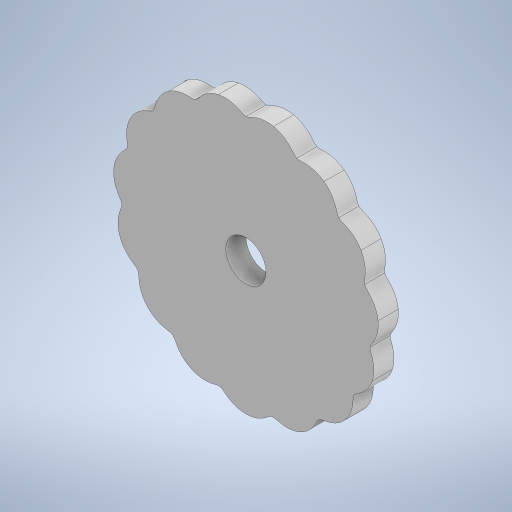
# Autodesk Inventor part: 사이클로이드 기어 001
Saved by Autodesk Inventor 2023 (Build 270158000, 158)
## iProperties
Created: 2022-06-19
Part Number: 사이클로이드 기어 001
Material: 일반
Document SubType Name: Modeling
Designer: fly01
Density: 1 g/cm^3
Appearance: 기본값
Author: fly01
Autodesk Inventor part; units mm, degrees
ref_plane "YZ Plane" through (0, 0, 0) normal (1, 0, 0) x (0, 1, 0)
ref_plane "XZ Plane" through (0, 0, 0) normal (0, 1, 0) x (-1, 0, 0)
ref_plane "XY Plane" through (0, 0, 0) normal (0, 0, 1) x (1, 0, 0)
sketch "스케치3" plane through (0, 0, 0) normal (0, 0, 1) x (1, 0, 0)
  circle A0 centre (0, 0) radius 30 construction
  circle A1 centre (-6.6532, 31.3007) radius 2 construction
  line L0 (-6.6532, 31.3007) -> (0, 0)
  line L1 (-6.6532, 31.3007) -> (-6.8611, 32.2789)
  line L2 (0, 30) -> (0, 0) construction
  spline S0 degree 4 poles (-6.8611, 32.2789) (-6.5216, 32.351) (-6.042, 32.4243) (-5.4252, 32.4676) (-4.6868, 32.4443) (-4.17, 32.3935) (-3.6752, 32.3125) (-3.207, 32.206) (-2.7688, 32.0793) (-2.3631, 31.9383) (-1.9912, 31.7892) (-1.6533, 31.6383) (-1.3481, 31.4918) (-1.0733, 31.3555) (-0.8255, 31.2347) (-0.5247, 31.1005) (-0.2949, 31.0253) (-0.1215, 30.9997) (0, 31) knots 0 0 0 0 0 0.166435 0.232217 0.297206 0.361177 0.423904 0.485164 0.544737 0.602405 0.657962 0.711221 0.762021 0.810262 0.855937 0.899201 1 1 1 1 1
  spline S1 degree 4 poles (-6.8611, 32.2789) (-7.2006, 32.2067) (-7.6685, 32.0786) (-8.2496, 31.8673) (-8.9146, 31.5456) (-9.3662, 31.289) (-9.7852, 31.0138) (-10.1697, 30.7261) (-10.5184, 30.4321) (-10.8317, 30.1383) (-11.1107, 29.8508) (-11.3581, 29.5755) (-11.5773, 29.3175) (-11.7729, 29.0812) (-11.9502, 28.8701) (-12.1704, 28.6252) (-12.3497, 28.463) (-12.4978, 28.3691) (-12.6088, 28.3199) knots 0 0 0 0 0 0.166435 0.232217 0.297206 0.361177 0.423904 0.485164 0.544737 0.602405 0.657962 0.711221 0.762021 0.810262 0.855937 0.899201 1 1 1 1 1
  spline S2 degree 4 poles (-19.3969, 26.6976) (-19.6777, 26.4935) (-20.0531, 26.1862) (-20.498, 25.7568) (-20.9747, 25.1925) (-21.2828, 24.7744) (-21.5537, 24.3525) (-21.7879, 23.9333) (-21.9869, 23.5229) (-22.1536, 23.1271) (-22.2916, 22.7509) (-22.4056, 22.3988) (-22.5009, 22.0739) (-22.5835, 21.7785) (-22.6595, 21.5135) (-22.7611, 21.2002) (-22.859, 20.9792) (-22.956, 20.8331) (-23.0375, 20.743) knots 0 0 0 0 0 0.166435 0.232217 0.297206 0.361177 0.423904 0.485164 0.544737 0.602405 0.657962 0.711221 0.762021 0.810262 0.855937 0.899201 1 1 1 1 1
  spline S3 degree 4 poles (-19.3969, 26.6976) (-19.1161, 26.9016) (-18.7078, 27.1636) (-18.1619, 27.454) (-17.4779, 27.733) (-16.9851, 27.8969) (-16.5002, 28.0241) (-16.0291, 28.1173) (-15.5773, 28.1798) (-15.1493, 28.2159) (-14.7489, 28.231) (-14.3788, 28.2306) (-14.0404, 28.2209) (-13.7339, 28.2081) (-13.4584, 28.1986) (-13.1291, 28.1984) (-12.8886, 28.2231) (-12.7197, 28.2703) (-12.6088, 28.3199) knots 0 0 0 0 0 0.166435 0.232217 0.297206 0.361177 0.423904 0.485164 0.544737 0.602405 0.657962 0.711221 0.762021 0.810262 0.855937 0.899201 1 1 1 1 1
  spline S4 degree 4 poles (-28.5788, 16.5) (-28.7524, 16.1994) (-28.9703, 15.766) (-29.2021, 15.1927) (-29.408, 14.4833) (-29.5195, 13.976) (-29.5954, 13.4804) (-29.6388, 13.0022) (-29.6537, 12.5463) (-29.6449, 12.117) (-29.618, 11.7172) (-29.5789, 11.3491) (-29.5339, 11.0136) (-29.4892, 10.7102) (-29.4509, 10.4371) (-29.4162, 10.1096) (-29.4157, 9.8678) (-29.445, 9.695) (-29.4828, 9.5795) knots 0 0 0 0 0 0.166435 0.232217 0.297206 0.361177 0.423904 0.485164 0.544737 0.602405 0.657962 0.711221 0.762021 0.810262 0.855937 0.899201 1 1 1 1 1
  spline S5 degree 4 poles (-28.5788, 16.5) (-28.4053, 16.8006) (-28.1389, 17.206) (-27.7583, 17.6934) (-27.2469, 18.2265) (-26.8633, 18.5766) (-26.4721, 18.8901) (-26.0796, 19.1668) (-25.6923, 19.4076) (-25.316, 19.6148) (-24.9564, 19.7913) (-24.6181, 19.9415) (-24.305, 20.0703) (-24.0199, 20.1833) (-23.7643, 20.2866) (-23.4633, 20.4204) (-23.2537, 20.5408) (-23.1186, 20.6526) (-23.0375, 20.743) knots 0 0 0 0 0 0.166435 0.232217 0.297206 0.361177 0.423904 0.485164 0.544737 0.602405 0.657962 0.711221 0.762021 0.810262 0.855937 0.899201 1 1 1 1 1
  spline S6 degree 4 poles (-32.8192, 3.4494) (-32.8555, 3.1042) (-32.8783, 2.6197) (-32.8569, 2.0017) (-32.7565, 1.2698) (-32.6519, 0.7611) (-32.5197, 0.2775) (-32.3648, -0.177) (-32.193, -0.5996) (-32.0104, -0.9883) (-31.8232, -1.3425) (-31.6378, -1.6629) (-31.4602, -1.9511) (-31.2959, -2.2101) (-31.1499, -2.4439) (-30.985, -2.7291) (-30.8862, -2.9497) (-30.8426, -3.1196) (-30.8302, -3.2404) knots 0 0 0 0 0 0.166435 0.232217 0.297206 0.361177 0.423904 0.485164 0.544737 0.602405 0.657962 0.711221 0.762021 0.810262 0.855937 0.899201 1 1 1 1 1
  spline S7 degree 4 poles (-32.8192, 3.4494) (-32.7829, 3.7946) (-32.7045, 4.2734) (-32.555, 4.8734) (-32.3047, 5.5684) (-32.0966, 6.0443) (-31.8668, 6.4898) (-31.6208, 6.9022) (-31.3649, 7.2798) (-31.1054, 7.622) (-30.8487, 7.9296) (-30.6007, 8.2044) (-30.367, 8.4494) (-30.1525, 8.6686) (-29.961, 8.867) (-29.7405, 9.1116) (-29.598, 9.3069) (-29.52, 9.4639) (-29.4828, 9.5795) knots 0 0 0 0 0 0.166435 0.232217 0.297206 0.361177 0.423904 0.485164 0.544737 0.602405 0.657962 0.711221 0.762021 0.810262 0.855937 0.899201 1 1 1 1 1
  spline S8 degree 4 poles (-31.3849, -10.1976) (-31.2776, -10.5277) (-31.1013, -10.9796) (-30.8304, -11.5355) (-30.441, -12.1632) (-30.1386, -12.5855) (-29.8211, -12.9735) (-29.4947, -13.3257) (-29.1659, -13.6418) (-28.841, -13.9226) (-28.5259, -14.1701) (-28.2262, -14.3874) (-27.9467, -14.5784) (-27.6913, -14.7482) (-27.4628, -14.9025) (-27.1962, -15.0959) (-27.0162, -15.2573) (-26.9073, -15.3947) (-26.8468, -15.5) knots 0 0 0 0 0 0.166435 0.232217 0.297206 0.361177 0.423904 0.485164 0.544737 0.602405 0.657962 0.711221 0.762021 0.810262 0.855937 0.899201 1 1 1 1 1
  spline S9 degree 4 poles (-31.3849, -10.1976) (-31.4921, -9.8675) (-31.6151, -9.3982) (-31.7227, -8.7892) (-31.7766, -8.0525) (-31.7802, -7.5332) (-31.7514, -7.0326) (-31.6944, -6.5559) (-31.6142, -6.1068) (-31.5163, -5.6886) (-31.4069, -5.3032) (-31.2922, -4.9513) (-31.1784, -4.6325) (-31.0715, -4.345) (-30.9773, -4.0859) (-30.8753, -3.7727) (-30.8246, -3.5363) (-30.8172, -3.3611) (-30.8302, -3.2404) knots 0 0 0 0 0 0.166435 0.232217 0.297206 0.361177 0.423904 0.485164 0.544737 0.602405 0.657962 0.711221 0.762021 0.810262 0.855937 0.899201 1 1 1 1 1
  spline S10 degree 4 poles (-24.5238, -22.0813) (-24.2915, -22.3392) (-23.9466, -22.6804) (-23.473, -23.078) (-22.862, -23.4931) (-22.414, -23.7558) (-21.9661, -23.9812) (-21.5247, -24.1702) (-21.0958, -24.3253) (-20.6847, -24.4496) (-20.2962, -24.5476) (-19.934, -24.6242) (-19.601, -24.685) (-19.2986, -24.7362) (-19.0271, -24.7842) (-18.7049, -24.8525) (-18.4748, -24.9267) (-18.3195, -25.0079) (-18.2213, -25.0795) knots 0 0 0 0 0 0.166435 0.232217 0.297206 0.361177 0.423904 0.485164 0.544737 0.602405 0.657962 0.711221 0.762021 0.810262 0.855937 0.899201 1 1 1 1 1
  spline S11 degree 4 poles (-24.5238, -22.0813) (-24.756, -21.8234) (-25.0593, -21.4447) (-25.4052, -20.9321) (-25.7542, -20.2811) (-25.9686, -19.808) (-26.1459, -19.3391) (-26.2878, -18.8803) (-26.3971, -18.4375) (-26.4778, -18.0157) (-26.5346, -17.6191) (-26.5729, -17.2509) (-26.5987, -16.9133) (-26.618, -16.6073) (-26.6373, -16.3322) (-26.6715, -16.0047) (-26.7213, -15.7681) (-26.7858, -15.6051) (-26.8468, -15.5) knots 0 0 0 0 0 0.166435 0.232217 0.297206 0.361177 0.423904 0.485164 0.544737 0.602405 0.657962 0.711221 0.762021 0.810262 0.855937 0.899201 1 1 1 1 1
  spline S12 degree 4 poles (-13.4223, -30.147) (-13.1052, -30.2882) (-12.6514, -30.4596) (-12.057, -30.6302) (-11.33, -30.7609) (-10.8138, -30.8186) (-10.313, -30.8423) (-9.8329, -30.8355) (-9.378, -30.8027) (-8.9518, -30.7491) (-8.5571, -30.6805) (-8.1951, -30.6032) (-7.8661, -30.5233) (-7.569, -30.4471) (-7.3015, -30.3805) (-6.9794, -30.3118) (-6.739, -30.286) (-6.564, -30.2971) (-6.4453, -30.3226) knots 0 0 0 0 0 0.166435 0.232217 0.297206 0.361177 0.423904 0.485164 0.544737 0.602405 0.657962 0.711221 0.762021 0.810262 0.855937 0.899201 1 1 1 1 1
  spline S13 degree 4 poles (-13.4223, -30.147) (-13.7394, -30.0058) (-14.1704, -29.7832) (-14.6949, -29.4557) (-15.2785, -29.0028) (-15.6668, -28.6579) (-16.0195, -28.3016) (-16.3357, -27.9402) (-16.6158, -27.5802) (-16.8611, -27.2277) (-17.0743, -26.8884) (-17.259, -26.5677) (-17.4198, -26.2698) (-17.562, -25.998) (-17.6915, -25.7546) (-17.856, -25.4693) (-17.9976, -25.2734) (-18.1229, -25.1507) (-18.2213, -25.0795) knots 0 0 0 0 0 0.166435 0.232217 0.297206 0.361177 0.423904 0.485164 0.544737 0.602405 0.657962 0.711221 0.762021 0.810262 0.855937 0.899201 1 1 1 1 1
  spline S14 degree 4 poles (0, -33) (0.3471, -33) (0.8314, -32.972) (1.4438, -32.8861) (2.1611, -32.7097) (2.6561, -32.5526) (3.1233, -32.3706) (3.5591, -32.169) (3.9614, -31.954) (4.3289, -31.7317) (4.6616, -31.5085) (4.9608, -31.2907) (5.2289, -31.0839) (5.4693, -30.8935) (5.6866, -30.7238) (5.9529, -30.53) (6.1621, -30.4087) (6.3264, -30.3476) (6.4453, -30.3226) knots 0 0 0 0 0 0.166435 0.232217 0.297206 0.361177 0.423904 0.485164 0.544737 0.602405 0.657962 0.711221 0.762021 0.810262 0.855937 0.899201 1 1 1 1 1
  spline S15 degree 4 poles (0, -33) (-0.3471, -33) (-0.8314, -32.972) (-1.4438, -32.8861) (-2.1611, -32.7097) (-2.6561, -32.5526) (-3.1233, -32.3706) (-3.5591, -32.169) (-3.9614, -31.954) (-4.3289, -31.7317) (-4.6616, -31.5085) (-4.9608, -31.2907) (-5.2289, -31.0839) (-5.4693, -30.8935) (-5.6866, -30.7238) (-5.9529, -30.53) (-6.1621, -30.4087) (-6.3264, -30.3476) (-6.4453, -30.3226) knots 0 0 0 0 0 0.166435 0.232217 0.297206 0.361177 0.423904 0.485164 0.544737 0.602405 0.657962 0.711221 0.762021 0.810262 0.855937 0.899201 1 1 1 1 1
  spline S16 degree 4 poles (13.4223, -30.147) (13.7394, -30.0058) (14.1704, -29.7832) (14.6949, -29.4557) (15.2785, -29.0028) (15.6668, -28.6579) (16.0195, -28.3016) (16.3357, -27.9402) (16.6158, -27.5802) (16.8611, -27.2277) (17.0743, -26.8884) (17.259, -26.5677) (17.4198, -26.2698) (17.562, -25.998) (17.6915, -25.7546) (17.856, -25.4693) (17.9976, -25.2734) (18.1229, -25.1507) (18.2213, -25.0795) knots 0 0 0 0 0 0.166435 0.232217 0.297206 0.361177 0.423904 0.485164 0.544737 0.602405 0.657962 0.711221 0.762021 0.810262 0.855937 0.899201 1 1 1 1 1
  spline S17 degree 4 poles (13.4223, -30.147) (13.1052, -30.2882) (12.6514, -30.4596) (12.057, -30.6302) (11.33, -30.7609) (10.8138, -30.8186) (10.313, -30.8423) (9.8329, -30.8355) (9.378, -30.8027) (8.9518, -30.7491) (8.5571, -30.6805) (8.1951, -30.6032) (7.8661, -30.5233) (7.569, -30.4471) (7.3015, -30.3805) (6.9794, -30.3118) (6.739, -30.286) (6.564, -30.2971) (6.4453, -30.3226) knots 0 0 0 0 0 0.166435 0.232217 0.297206 0.361177 0.423904 0.485164 0.544737 0.602405 0.657962 0.711221 0.762021 0.810262 0.855937 0.899201 1 1 1 1 1
  spline S18 degree 4 poles (24.5238, -22.0813) (24.756, -21.8234) (25.0593, -21.4447) (25.4052, -20.9321) (25.7542, -20.2811) (25.9686, -19.808) (26.1459, -19.3391) (26.2878, -18.8803) (26.3971, -18.4375) (26.4778, -18.0157) (26.5346, -17.6191) (26.5729, -17.2509) (26.5987, -16.9133) (26.618, -16.6073) (26.6373, -16.3322) (26.6715, -16.0047) (26.7213, -15.7681) (26.7858, -15.6051) (26.8468, -15.5) knots 0 0 0 0 0 0.166435 0.232217 0.297206 0.361177 0.423904 0.485164 0.544737 0.602405 0.657962 0.711221 0.762021 0.810262 0.855937 0.899201 1 1 1 1 1
  spline S19 degree 4 poles (24.5238, -22.0813) (24.2915, -22.3392) (23.9466, -22.6804) (23.473, -23.078) (22.862, -23.4931) (22.414, -23.7558) (21.9661, -23.9812) (21.5247, -24.1702) (21.0958, -24.3253) (20.6847, -24.4496) (20.2962, -24.5476) (19.934, -24.6242) (19.601, -24.685) (19.2986, -24.7362) (19.0271, -24.7842) (18.7049, -24.8525) (18.4748, -24.9267) (18.3195, -25.0079) (18.2213, -25.0795) knots 0 0 0 0 0 0.166435 0.232217 0.297206 0.361177 0.423904 0.485164 0.544737 0.602405 0.657962 0.711221 0.762021 0.810262 0.855937 0.899201 1 1 1 1 1
  spline S20 degree 4 poles (31.3849, -10.1976) (31.4921, -9.8675) (31.6151, -9.3982) (31.7227, -8.7892) (31.7766, -8.0525) (31.7802, -7.5332) (31.7514, -7.0326) (31.6944, -6.5559) (31.6142, -6.1068) (31.5163, -5.6886) (31.4069, -5.3032) (31.2922, -4.9513) (31.1784, -4.6325) (31.0715, -4.345) (30.9773, -4.0859) (30.8753, -3.7727) (30.8246, -3.5363) (30.8172, -3.3611) (30.8302, -3.2404) knots 0 0 0 0 0 0.166435 0.232217 0.297206 0.361177 0.423904 0.485164 0.544737 0.602405 0.657962 0.711221 0.762021 0.810262 0.855937 0.899201 1 1 1 1 1
  spline S21 degree 4 poles (31.3849, -10.1976) (31.2776, -10.5277) (31.1013, -10.9796) (30.8304, -11.5355) (30.441, -12.1632) (30.1386, -12.5855) (29.8211, -12.9735) (29.4947, -13.3257) (29.1659, -13.6418) (28.841, -13.9226) (28.5259, -14.1701) (28.2262, -14.3874) (27.9467, -14.5784) (27.6913, -14.7482) (27.4628, -14.9025) (27.1962, -15.0959) (27.0162, -15.2573) (26.9073, -15.3947) (26.8468, -15.5) knots 0 0 0 0 0 0.166435 0.232217 0.297206 0.361177 0.423904 0.485164 0.544737 0.602405 0.657962 0.711221 0.762021 0.810262 0.855937 0.899201 1 1 1 1 1
  spline S22 degree 4 poles (32.8192, 3.4494) (32.7829, 3.7946) (32.7045, 4.2734) (32.555, 4.8734) (32.3047, 5.5684) (32.0966, 6.0443) (31.8668, 6.4898) (31.6208, 6.9022) (31.3649, 7.2798) (31.1054, 7.622) (30.8487, 7.9296) (30.6007, 8.2044) (30.367, 8.4494) (30.1525, 8.6686) (29.961, 8.867) (29.7405, 9.1116) (29.598, 9.3069) (29.52, 9.4639) (29.4828, 9.5795) knots 0 0 0 0 0 0.166435 0.232217 0.297206 0.361177 0.423904 0.485164 0.544737 0.602405 0.657962 0.711221 0.762021 0.810262 0.855937 0.899201 1 1 1 1 1
  spline S23 degree 4 poles (32.8192, 3.4494) (32.8555, 3.1042) (32.8783, 2.6197) (32.8569, 2.0017) (32.7565, 1.2698) (32.6519, 0.7611) (32.5197, 0.2775) (32.3648, -0.177) (32.193, -0.5996) (32.0104, -0.9883) (31.8232, -1.3425) (31.6378, -1.6629) (31.4602, -1.9511) (31.2959, -2.2101) (31.1499, -2.4439) (30.985, -2.7291) (30.8862, -2.9497) (30.8426, -3.1196) (30.8302, -3.2404) knots 0 0 0 0 0 0.166435 0.232217 0.297206 0.361177 0.423904 0.485164 0.544737 0.602405 0.657962 0.711221 0.762021 0.810262 0.855937 0.899201 1 1 1 1 1
  spline S24 degree 4 poles (28.5788, 16.5) (28.4053, 16.8006) (28.1389, 17.206) (27.7583, 17.6934) (27.2469, 18.2265) (26.8633, 18.5766) (26.4721, 18.8901) (26.0796, 19.1668) (25.6923, 19.4076) (25.316, 19.6148) (24.9564, 19.7913) (24.6181, 19.9415) (24.305, 20.0703) (24.0199, 20.1833) (23.7643, 20.2866) (23.4633, 20.4204) (23.2537, 20.5408) (23.1186, 20.6526) (23.0375, 20.743) knots 0 0 0 0 0 0.166435 0.232217 0.297206 0.361177 0.423904 0.485164 0.544737 0.602405 0.657962 0.711221 0.762021 0.810262 0.855937 0.899201 1 1 1 1 1
  spline S25 degree 4 poles (28.5788, 16.5) (28.7524, 16.1994) (28.9703, 15.766) (29.2021, 15.1927) (29.408, 14.4833) (29.5195, 13.976) (29.5954, 13.4804) (29.6388, 13.0022) (29.6537, 12.5463) (29.6449, 12.117) (29.618, 11.7172) (29.5789, 11.3491) (29.5339, 11.0136) (29.4892, 10.7102) (29.4509, 10.4371) (29.4162, 10.1096) (29.4157, 9.8678) (29.445, 9.695) (29.4828, 9.5795) knots 0 0 0 0 0 0.166435 0.232217 0.297206 0.361177 0.423904 0.485164 0.544737 0.602405 0.657962 0.711221 0.762021 0.810262 0.855937 0.899201 1 1 1 1 1
  spline S26 degree 4 poles (19.3969, 26.6976) (19.1161, 26.9016) (18.7078, 27.1636) (18.1619, 27.454) (17.4779, 27.733) (16.9851, 27.8969) (16.5002, 28.0241) (16.0291, 28.1173) (15.5773, 28.1798) (15.1493, 28.2159) (14.7489, 28.231) (14.3788, 28.2306) (14.0404, 28.2209) (13.7339, 28.2081) (13.4584, 28.1986) (13.1291, 28.1984) (12.8886, 28.2231) (12.7197, 28.2703) (12.6088, 28.3199) knots 0 0 0 0 0 0.166435 0.232217 0.297206 0.361177 0.423904 0.485164 0.544737 0.602405 0.657962 0.711221 0.762021 0.810262 0.855937 0.899201 1 1 1 1 1
  spline S27 degree 4 poles (19.3969, 26.6976) (19.6777, 26.4935) (20.0531, 26.1862) (20.498, 25.7568) (20.9747, 25.1925) (21.2828, 24.7744) (21.5537, 24.3525) (21.7879, 23.9333) (21.9869, 23.5229) (22.1536, 23.1271) (22.2916, 22.7509) (22.4056, 22.3988) (22.5009, 22.0739) (22.5835, 21.7785) (22.6595, 21.5135) (22.7611, 21.2002) (22.859, 20.9792) (22.956, 20.8331) (23.0375, 20.743) knots 0 0 0 0 0 0.166435 0.232217 0.297206 0.361177 0.423904 0.485164 0.544737 0.602405 0.657962 0.711221 0.762021 0.810262 0.855937 0.899201 1 1 1 1 1
  spline S28 degree 4 poles (6.8611, 32.2789) (6.5216, 32.351) (6.042, 32.4243) (5.4252, 32.4676) (4.6868, 32.4443) (4.17, 32.3935) (3.6752, 32.3125) (3.207, 32.206) (2.7688, 32.0793) (2.3631, 31.9383) (1.9912, 31.7892) (1.6533, 31.6383) (1.3481, 31.4918) (1.0733, 31.3555) (0.8255, 31.2347) (0.5247, 31.1005) (0.2949, 31.0253) (0.1215, 30.9997) (0, 31) knots 0 0 0 0 0 0.166435 0.232217 0.297206 0.361177 0.423904 0.485164 0.544737 0.602405 0.657962 0.711221 0.762021 0.810262 0.855937 0.899201 1 1 1 1 1
  spline S29 degree 4 poles (6.8611, 32.2789) (7.2006, 32.2067) (7.6685, 32.0786) (8.2496, 31.8673) (8.9146, 31.5456) (9.3662, 31.289) (9.7852, 31.0138) (10.1697, 30.7261) (10.5184, 30.4321) (10.8317, 30.1383) (11.1107, 29.8508) (11.3581, 29.5755) (11.5773, 29.3175) (11.7729, 29.0812) (11.9502, 28.8701) (12.1704, 28.6252) (12.3497, 28.463) (12.4978, 28.3691) (12.6088, 28.3199) knots 0 0 0 0 0 0.166435 0.232217 0.297206 0.361177 0.423904 0.485164 0.544737 0.602405 0.657962 0.711221 0.762021 0.810262 0.855937 0.899201 1 1 1 1 1
  circle A2 centre (0, 0) radius 5
  point P0 (-0.1872, 31.0151)
  point P1 (-0.3808, 31.0599)
  point P2 (-0.5869, 31.1325)
  point P3 (-0.8111, 31.23)
  point P4 (-1.0585, 31.3487)
  point P5 (-1.3334, 31.4837)
  point P6 (-1.6391, 31.6295)
  point P7 (-1.9777, 31.7801)
  point P8 (-2.3504, 31.9292)
  point P9 (-2.757, 32.0704)
  point P10 (-3.1962, 32.1974)
  point P11 (-3.6655, 32.3042)
  point P12 (-4.1615, 32.3855)
  point P13 (-4.6797, 32.4365)
  point P14 (-5.2147, 32.4535)
  point P15 (-5.7609, 32.4338)
  point P16 (-6.3118, 32.3757)
  point P17 (-12.4439, 28.4099)
  point P18 (-12.2853, 28.5295)
  point P19 (-12.1266, 28.6796)
  point P20 (-11.9614, 28.86)
  point P21 (-11.7837, 29.069)
  point P22 (-11.5874, 29.3041)
  point P23 (-11.3675, 29.5616)
  point P24 (-11.1194, 29.837)
  point P25 (-10.8396, 30.1248)
  point P26 (-10.5256, 30.4192)
  point P27 (-10.176, 30.7138)
  point P28 (-9.7907, 31.0023)
  point P29 (-9.3706, 31.2783)
  point P30 (-8.918, 31.5356)
  point P31 (-8.4362, 31.7688)
  point P32 (-7.9292, 31.9729)
  point P33 (-7.4023, 32.144)
  point P34 (-19.8364, 26.3542)
  point P35 (-20.2483, 25.9836)
  point P36 (-20.6284, 25.591)
  point P37 (-20.9737, 25.1819)
  point P38 (-21.2825, 24.7627)
  point P39 (-21.554, 24.3398)
  point P40 (-21.7887, 23.9195)
  point P41 (-21.9882, 23.5081)
  point P42 (-22.1553, 23.1115)
  point P43 (-22.2939, 22.7348)
  point P44 (-22.4085, 22.3823)
  point P45 (-22.5047, 22.0576)
  point P46 (-22.5883, 21.763)
  point P47 (-22.6657, 21.4997)
  point P48 (-22.7432, 21.2678)
  point P49 (-22.8272, 21.0661)
  point P50 (-22.9234, 20.8923)
  point P51 (-18.9345, 27.0095)
  point P52 (-18.4548, 27.2866)
  point P53 (-17.9639, 27.5268)
  point P54 (-17.4682, 27.7288)
  point P55 (-16.9741, 27.893)
  point P56 (-16.4879, 28.0205)
  point P57 (-16.0157, 28.1138)
  point P58 (-15.5628, 28.1764)
  point P59 (-15.134, 28.2128)
  point P60 (-14.7329, 28.2282)
  point P61 (-14.3622, 28.2283)
  point P62 (-14.0237, 28.2194)
  point P63 (-13.7177, 28.2079)
  point P64 (-13.4434, 28.2002)
  point P65 (-13.1988, 28.2022)
  point P66 (-12.9811, 28.2197)
  point P67 (-12.786, 28.2576)
  point P68 (-28.8407, 16.0075)
  point P69 (-29.0662, 15.5015)
  point P70 (-29.2537, 14.9882)
  point P71 (-29.4029, 14.474)
  point P72 (-29.5145, 13.9655)
  point P73 (-29.5904, 13.4687)
  point P74 (-29.6339, 12.9893)
  point P75 (-29.6488, 12.5324)
  point P76 (-29.6402, 12.102)
  point P77 (-29.6135, 11.7015)
  point P78 (-29.5749, 11.3329)
  point P79 (-29.5307, 10.9971)
  point P80 (-29.4873, 10.694)
  point P81 (-29.4509, 10.422)
  point P82 (-29.4274, 10.1786)
  point P83 (-29.422, 9.9602)
  point P84 (-29.4393, 9.7623)
  point P85 (-28.2833, 16.973)
  point P86 (-27.9578, 17.4213)
  point P87 (-27.607, 17.8404)
  point P88 (-27.2363, 18.2266)
  point P89 (-26.8517, 18.5775)
  point P90 (-26.4594, 18.8917)
  point P91 (-26.066, 19.1691)
  point P92 (-25.6778, 19.4105)
  point P93 (-25.3008, 19.6181)
  point P94 (-24.9406, 19.7953)
  point P95 (-24.602, 19.9462)
  point P96 (-24.2892, 20.0758)
  point P97 (-24.0049, 20.1897)
  point P98 (-23.7512, 20.2942)
  point P99 (-23.5286, 20.3956)
  point P100 (-23.3368, 20.5001)
  point P101 (-23.174, 20.614)
  point P102 (-32.8582, 2.893)
  point P103 (-32.8583, 2.339)
  point P104 (-32.8208, 1.7938)
  point P105 (-32.748, 1.2635)
  point P106 (-32.6431, 0.7535)
  point P107 (-32.5104, 0.2687)
  point P108 (-32.3551, -0.1869)
  point P109 (-32.1829, -0.6104)
  point P110 (-32, -1)
  point P111 (-31.8127, -1.355)
  point P112 (-31.6275, -1.6761)
  point P113 (-31.4506, -1.9648)
  point P114 (-31.2876, -2.2241)
  point P115 (-31.1437, -2.4578)
  point P116 (-31.0233, -2.6706)
  point P117 (-30.9295, -2.8679)
  point P118 (-30.8648, -3.0558)
  point P119 (-32.7416, 4.0018)
  point P120 (-32.6266, 4.5437)
  point P121 (-32.4766, 5.0692)
  point P122 (-32.2951, 5.5728)
  point P123 (-32.0864, 6.0498)
  point P124 (-31.8559, 6.4964)
  point P125 (-31.6092, 6.9098)
  point P126 (-31.3527, 7.2883)
  point P127 (-31.0928, 7.6313)
  point P128 (-30.8358, 7.9397)
  point P129 (-30.5879, 8.2152)
  point P130 (-30.3548, 8.4608)
  point P131 (-30.1415, 8.6806)
  point P132 (-29.9522, 8.8792)
  point P133 (-29.7901, 9.0623)
  point P134 (-29.6574, 9.2358)
  point P135 (-29.555, 9.4061)
  point P136 (-31.1941, -10.7217)
  point P137 (-30.9689, -11.2279)
  point P138 (-30.713, -11.7107)
  point P139 (-30.4307, -12.1656)
  point P140 (-30.1274, -12.5888)
  point P141 (-29.8091, -12.9777)
  point P142 (-29.4819, -13.3307)
  point P143 (-29.1523, -13.6476)
  point P144 (-28.8267, -13.9291)
  point P145 (-28.5112, -14.1773)
  point P146 (-28.2115, -14.3953)
  point P147 (-27.9324, -14.5871)
  point P148 (-27.678, -14.7577)
  point P149 (-27.4515, -14.9126)
  point P150 (-27.2549, -15.058)
  point P151 (-27.089, -15.2001)
  point P152 (-26.9535, -15.3454)
  point P153 (-31.5386, -9.6614)
  point P154 (-31.654, -9.1196)
  point P155 (-31.7307, -8.5785)
  point P156 (-31.7697, -8.0446)
  point P157 (-31.7731, -7.5239)
  point P158 (-31.7441, -7.0222)
  point P159 (-31.6869, -6.5442)
  point P160 (-31.6066, -6.0942)
  point P161 (-31.5086, -5.675)
  point P162 (-31.3993, -5.2888)
  point P163 (-31.2849, -4.9363)
  point P164 (-31.1718, -4.617)
  point P165 (-31.0663, -4.3295)
  point P166 (-30.9742, -4.0711)
  point P167 (-30.9006, -3.8379)
  point P168 (-30.8499, -3.6254)
  point P169 (-30.8256, -3.4282)
  point P170 (-24.1363, -22.4825)
  point P171 (-23.7248, -22.8534)
  point P172 (-23.2945, -23.1903)
  point P173 (-22.8516, -23.4911)
  point P174 (-22.4024, -23.7543)
  point P175 (-21.9534, -23.9801)
  point P176 (-21.5109, -24.1696)
  point P177 (-21.081, -24.325)
  point P178 (-20.669, -24.4498)
  point P179 (-20.2799, -24.5482)
  point P180 (-19.9174, -24.6254)
  point P181 (-19.5844, -24.6871)
  point P182 (-19.2827, -24.7395)
  point P183 (-19.0127, -24.7889)
  point P184 (-18.774, -24.8417)
  point P185 (-18.5646, -24.9041)
  point P186 (-18.3817, -24.9817)
  point P187 (-24.8823, -21.6541)
  point P188 (-25.2081, -21.206)
  point P189 (-25.4982, -20.7429)
  point P190 (-25.751, -20.271)
  point P191 (-25.9659, -19.7967)
  point P192 (-26.1435, -19.3266)
  point P193 (-26.2857, -18.8667)
  point P194 (-26.3953, -18.4228)
  point P195 (-26.4763, -18.0001)
  point P196 (-26.5335, -17.6028)
  point P197 (-26.5724, -17.2342)
  point P198 (-26.599, -16.8966)
  point P199 (-26.6195, -16.591)
  dimension "d15" = 60
  dimension "d16" = 4
  dimension "d17" = 1
  dimension "d19" = 180
  dimension "d20" = 12
  dimension "d23" = 360
  dimension "d27" = 10
  constraints: 18 symmetric about line, 6 end point, 2 centre point, 2 coincident, 1 vertical, 1 vertical alignment, 1159 other
  measures "d16" diameter of A1
  measures "d17" distance of L0.start L1.end
  measures "d19" angle of L1 L0
  measures "d20" angle of L2 L0
  measures "d27" diameter of A2
extrude "돌출3" add sketch "스케치3" along normal blind 5
equation "\"d20\" = 0.0666667 * d19"
